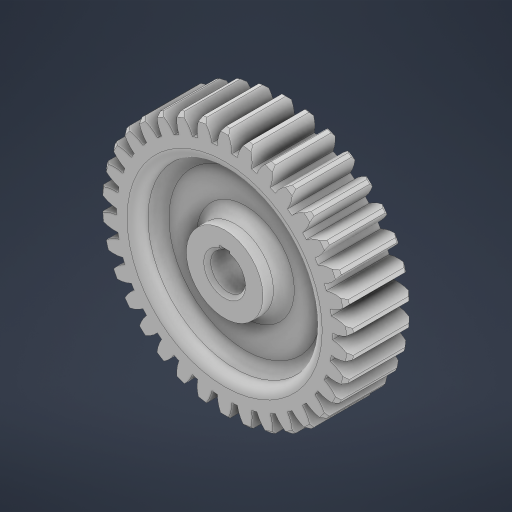
# Autodesk Inventor part: 부품4
Saved by Autodesk Inventor 2023 (Build 270158000, 158)
## iProperties
Created: 2022-11-14
Part Number: 부품4
Material: 일반
Document SubType Name: Modeling
Designer: LJH
Density: 1 g/cm^3
Appearance: 기본값
Author: LJH
Autodesk Inventor part; units mm, degrees
ref_plane "YZ Plane" through (0, 0, 0) normal (1, 0, 0) x (0, 1, 0)
ref_plane "XZ Plane" through (0, 0, 0) normal (0, 1, 0) x (-1, 0, 0)
ref_plane "XY Plane" through (0, 0, 0) normal (0, 0, 1) x (1, 0, 0)
sketch "스케치1" plane through (0, 0, 0) normal (0, 0, 1) x (1, 0, 0)
  circle A0 centre (0, 0) radius 34
  circle A1 centre (0, 0) radius 36
  circle A2 centre (0, 0) radius 31
  dimension "d2" = 68
  dimension "d27" = 72
  dimension "d28" = 5
  constraints: 3 centre point, 2 coincident
  measures "d2" diameter of A0
  measures "d27" diameter of A1
  measures "d28" radial gap between concentric circles of A1 A2
extrude "돌출1" add sketch "스케치1" along normal mid plane 18 contours A2
sketch "스케치2" plane through (0, 0, 0) normal (1, 0, 0) x (0, 1, 0)
  line L0 (40.7313, 0) -> (0, 0)
  line L1 (25, 9) -> (11, 9)
  line L2 (11, 9) -> (11, 3)
  line L3 (11, 3) -> (25, 3)
  line L4 (25, 3) -> (25, 9)
  line L5 (25, -9) -> (11, -9)
  line L6 (11, -9) -> (11, -3)
  line L7 (25, -3) -> (25, -9)
  line L8 (25, -3) -> (11, -3)
  line L9 (0, -12.6) -> (0, 12.6) projected
  point P0 (34, 9)
  point P1 (-34, 9)
  point P2 (11, 6)
  point P3 (11, -6)
  dimension "d3" = 11
  dimension "d4" = 14
  dimension "d5" = 6
  constraints: 18 end point, 5 symmetric about line, 2 horizontal, 2 parallel, 2 perpendicular, 1 midpoint
  measures "d3" horizontal distance of L0.end point (11, 6)
  measures "d4" distance between parallel lines of L2 L4
  measures "d5" distance between parallel lines of L3 L8
revolve "회전1" cut sketch "스케치2" angle 360 about axis through (0, 0, -10) along (0, 0, -1)
sketch "스케치3" plane through (0, 0, 9) normal (0, 0, 1) x (1, 0, 0)
  circle A0 centre (0, 0) radius 5
  line L0 (-1.5, 6.4) -> (1.5, 6.4)
  line L1 (1.5, 6.4) -> (1.5, 2.1456)
  line L2 (1.5, 2.1456) -> (-1.5, 2.1456)
  line L3 (-1.5, 2.1456) -> (-1.5, 6.4)
  point P0 (0, 6.4)
  point P1 (0, -5)
  point P2 (-1.5, 4.7697)
  point P3 (1.5, 4.7697)
  dimension "d7" = 10
  dimension "d8" = 11.4
  dimension "d9" = 3
  constraints: 8 end point, 2 parallel, 1 coincident, 1 horizontal, 1 midpoint, 1 perpendicular, 1 vertical alignment, 3 other
  measures "d8" distance from line of point (0, -5) L0
  measures "d9" distance between parallel lines of L3 L1
extrude "돌출2" cut sketch "스케치3" against normal blind 18
fillet "모깎기1" radius 3 6 edges at (0, -11, -3) (0, -25, -3) (0, -25, -9) (0, -11, 3) (0, -25, 3) (0, -25, 9)
chamfer "모따기1" distance 1 angle 45 2 edges at (0, -5, 9) (0, -5, -9)
sketch "스케치4" plane through (0, 0, -9) normal (0, 0, -1) x (-1, 0, 0)
  circle A0 centre (0, 0) radius 36
  circle A1 centre (0, 0) radius 28 projected
  circle A2 centre (0, 0) radius 31
  circle A3 centre (0, 0) radius 34 projected
  line L0 (0, 0) -> (0, 40.018)
  line L1 (-1.57, 0) -> (-1.57, 40.018)
  line L2 (-0.57, 0) -> (-0.57, 40.018)
  line L3 (-2.07, 0) -> (-2.07, 40.018)
  arc A4 (-0.57, 35.9955) -> (-2.07, 30.9308) centre (7.0441, 30.986) ccw
  arc A5 (2.07, 30.9308) -> (0.57, 35.9955) centre (-7.0441, 30.986) ccw
  point P0 (2.07, 30.9308)
  point P1 (0.57, 35.9955)
  dimension "d16" = 72
  dimension "d21" = 5
  dimension "d22" = 1.57
  dimension "d23" = 1
  dimension "d24" = 0.5
  constraints: 8 end point, 4 point on circle, 3 parallel, 3 symmetric about line, 2 centre point, 2 point on line, 1 coincident, 1 vertical, 7 other
  measures "d22" distance between parallel lines of L0 L1
  measures "d23" distance between parallel lines of L1 L2
  measures "d24" distance between parallel lines of L1 L3
extrude "돌출3" add sketch "스케치4" against normal blind 18 contours A5 A3 L0 A0 | L0 A3 L2 A0 | A5 A2 L0 A3 | L2 A3 A4 | L0 A2 L2 A3 | A3 L2 A2 L1 | L1 A2 A4
chamfer "모따기2" distance 1 angle 45 2 edges at (0, 36, -9) (0, 36, 9)
pattern_circular "원형 패턴1" count 34 over 360 about axis through (0, 0, 0) along (0, 0, 1) of "돌출3", "모따기2"
